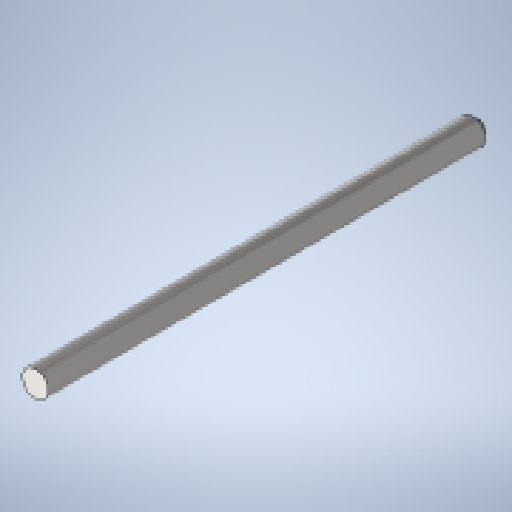
# Autodesk Inventor part: End Guides - Rail
Saved by Autodesk Inventor 2023.2 (Build 272271000, 271)
## iProperties
Created: 2024-02-24
Part Number: End Guides - Rail
Material: Stainless Steel
Document SubType Name: Modeling
Designer: Nathan Cai
Mass: 2.51359 g
Surface Area: 4.33069 cm^2
Volume: 0.314199 cm^3
Density: 8 g/cm^3
Appearance: Semi-Polished
Author: Nathan Cai
Autodesk Inventor part; units mm, degrees
ref_plane "YZ Plane" through (0, 0, 0) normal (1, 0, 0) x (0, 1, 0)
ref_plane "XZ Plane" through (0, 0, 0) normal (0, 1, 0) x (-1, 0, 0)
ref_plane "XY Plane" through (0, 0, 0) normal (0, 0, 1) x (1, 0, 0)
sketch "Sketch1" plane through (0, 0, 0) normal (0, 0, 1) x (1, 0, 0)
  circle A0 centre (0, 0) radius 1.5
  dimension "d0" = 3
  constraints: 1 centre point, 1 coincident
  measures "d0" diameter of A0
extrude "Extrusion1" add sketch "Sketch1" along normal blind 50.8
chamfer "Chamfer1" distance 0.5 angle 45 1 edges at (-1.5, 0, 0)
body "Solid1"
